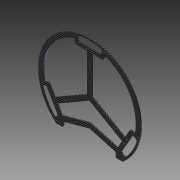
# Autodesk Inventor part: Middle Plate
Saved by Autodesk Inventor 2015 (Build 190159000, 159)
## iProperties
Created: 2016-08-09
Part Number: Middle Plate
Material: Polycarbonate, Clear
Document SubType Name: Modeling
Designer: James Yelland
Density: 1.2 g/cm^3
Appearance: Polycarbonate - Clear
Mass: 31.4673 g
Surface Area: 306.094 cm^2
Volume: 26.2228 cm^3
Author: James Yelland
Autodesk Inventor part; units mm, degrees
ref_plane "YZ Plane" through (0, 0, 0) normal (1, 0, 0) x (0, 1, 0)
ref_plane "XZ Plane" through (0, 0, 0) normal (0, 1, 0) x (-1, 0, 0)
ref_plane "XY Plane" through (0, 0, 0) normal (0, 0, 1) x (1, 0, 0)
sketch "Sketch1" plane through (0, 0, 0) normal (0, 1, 0) x (-1, 0, 0)
  circle A0 centre (-51.9527, -30.0153) radius 1.6
  circle A1 centre (0, 60) radius 1.6
  circle A2 centre (51.9527, -30.0153) radius 1.6
  line L0 (-76.2102, -44) -> (-65.7102, -62.1865)
  line L1 (-67.1743, -67.6506) -> (-69.6351, -69.0713)
  line L2 (-94.6351, -25.7701) -> (-92.1743, -24.3494)
  line L3 (-86.7102, -25.8135) -> (-76.2102, -44)
  arc A3 (-96.4496, -30.438) -> (-74.5849, -68.3088) centre (0, 0) ccw
  arc A4 (-94.6351, -25.7701) -> (-96.4496, -30.438) centre (-92.6351, -29.2342) ccw
  arc A5 (-86.7102, -25.8135) -> (-92.1743, -24.3494) centre (-90.1743, -27.8135) ccw
  arc A6 (-67.1743, -67.6506) -> (-65.7102, -62.1865) centre (-69.1743, -64.1865) ccw
  arc A7 (-74.5849, -68.3088) -> (-69.6351, -69.0713) centre (-71.6351, -65.6072) ccw
  line L4 (65.7102, -62.1865) -> (76.2102, -44)
  arc A8 (74.5849, -68.3088) -> (96.4496, -30.438) centre (0, 0) ccw
  arc A9 (65.7102, -62.1865) -> (67.1743, -67.6506) centre (69.1743, -64.1865) ccw
  line L5 (69.6351, -69.0713) -> (67.1743, -67.6506)
  arc A10 (69.6351, -69.0713) -> (74.5849, -68.3088) centre (71.6351, -65.6072) ccw
  arc A11 (92.1743, -24.3494) -> (86.7102, -25.8135) centre (90.1743, -27.8135) ccw
  line L6 (92.1743, -24.3494) -> (94.6351, -25.7701)
  arc A12 (96.4496, -30.438) -> (94.6351, -25.7701) centre (92.6351, -29.2342) ccw
  line L7 (76.2102, -44) -> (86.7102, -25.8135)
  line L8 (21, 88) -> (0, 88)
  arc A13 (21.8647, 98.7468) -> (-21.8647, 98.7468) centre (0, 0) ccw
  arc A14 (21, 88) -> (25, 92) centre (21, 92) ccw
  line L9 (25, 94.8414) -> (25, 92)
  arc A15 (25, 94.8414) -> (21.8647, 98.7468) centre (21, 94.8414) ccw
  arc A16 (-25, 92) -> (-21, 88) centre (-21, 92) ccw
  line L10 (-25, 92) -> (-25, 94.8414)
  arc A17 (-21.8647, 98.7468) -> (-25, 94.8414) centre (-21, 94.8414) ccw
  line L11 (0, 88) -> (-21, 88)
  line L12 (-75.1122, -39.9019) -> (-77.6122, -35.5718)
  line L13 (-77.6122, -35.5718) -> (-75.8801, -34.5718)
  line L14 (-75.8801, -34.5718) -> (-73.3801, -38.9019)
  line L15 (-73.3801, -38.9019) -> (-75.1122, -39.9019)
  line L16 (-70.3801, -44.0981) -> (-72.1122, -45.0981)
  line L17 (-67.8801, -48.4282) -> (-70.3801, -44.0981)
  line L18 (-69.6122, -49.4282) -> (-67.8801, -48.4282)
  line L19 (-72.1122, -45.0981) -> (-69.6122, -49.4282)
  line L20 (70.3801, -44.0981) -> (72.1122, -45.0981)
  line L21 (72.1122, -45.0981) -> (69.6122, -49.4282)
  line L22 (67.8801, -48.4282) -> (70.3801, -44.0981)
  line L23 (69.6122, -49.4282) -> (67.8801, -48.4282)
  line L24 (75.8801, -34.5718) -> (73.3801, -38.9019)
  line L25 (75.1122, -39.9019) -> (77.6122, -35.5718)
  line L26 (73.3801, -38.9019) -> (75.1122, -39.9019)
  line L27 (77.6122, -35.5718) -> (75.8801, -34.5718)
  line L28 (3, 83) -> (3, 85)
  line L29 (3, 85) -> (8, 85)
  line L30 (8, 83) -> (3, 83)
  line L31 (8, 85) -> (8, 83)
  line L32 (-8, 83) -> (-3, 83)
  line L33 (-3, 85) -> (-8, 85)
  line L34 (-3, 83) -> (-3, 85)
  line L35 (-8, 85) -> (-8, 83)
  line L36 (54.0074, -78) -> (54.0074, -71.5202)
  line L37 (52.5426, -69.5932) -> (0.5352, -55.1487)
  line L38 (-52.5426, -69.5932) -> (-0.5352, -55.1487)
  line L39 (-54.0074, -78) -> (-54.0074, -71.5202)
  arc A18 (68.5743, -79.5146) -> (-68.5743, -79.5146) centre (0, 0) ccw
  line L40 (67.2681, -80) -> (56.0074, -80)
  line L41 (-56.0074, -80) -> (-67.2681, -80)
  arc A19 (54.0074, -78) -> (56.0074, -80) centre (56.0074, -78) ccw
  arc A20 (67.2681, -80) -> (68.5743, -79.5146) centre (67.2681, -78) ccw
  arc A21 (54.0074, -71.5202) -> (52.5426, -69.5932) centre (52.0074, -71.5202) ccw
  arc A22 (0.5352, -55.1487) -> (-0.5352, -55.1487) centre (0, -57.0757) ccw
  arc A23 (-52.5426, -69.5932) -> (-54.0074, -71.5202) centre (-52.0074, -71.5202) ccw
  arc A24 (-56.0074, -80) -> (-54.0074, -78) centre (-56.0074, -78) ccw
  arc A25 (-68.5743, -79.5146) -> (-67.2681, -80) centre (-67.2681, -78) ccw
  line L42 (-30, 85) -> (-30, 87.3212)
  line L43 (30, 85) -> (30, 87.3212)
  arc A26 (-30, 85) -> (-25, 80) centre (-25, 85) ccw
  arc A27 (25, 80) -> (30, 85) centre (25, 85) ccw
  circle A28 centre (-30, 95.3939) radius 1.6
  circle A29 centre (30, 95.3939) radius 1.6
  arc A30 (-81.782, -18.3494) -> (-88.6122, -16.5192) centre (-86.1122, -20.8494) ccw
  line L44 (-88.6122, -16.5192) -> (-90.6224, -17.6799)
  circle A31 centre (-67.6136, -73.6777) radius 1.6
  circle A32 centre (-97.6136, -21.7162) radius 1.6
  arc A33 (88.6122, -16.5192) -> (81.782, -18.3494) centre (86.1122, -20.8494) ccw
  line L45 (88.6122, -16.5192) -> (90.6224, -17.6799)
  circle A34 centre (97.6136, -21.7162) radius 1.6
  circle A35 centre (67.6136, -73.6777) radius 1.6
  arc A36 (-32.6882, 89.1991) -> (-93.5928, -16.2908) centre (0, 0) ccw
  arc A37 (93.5928, -16.2908) -> (32.6882, 89.1991) centre (0, 0) ccw
  arc A38 (-30, 87.3212) -> (-32.6882, 89.1991) centre (-32, 87.3212) ccw
  arc A39 (32.6882, 89.1991) -> (30, 87.3212) centre (32, 87.3212) ccw
  arc A40 (90.6224, -17.6799) -> (93.5928, -16.2908) centre (91.6224, -15.9478) ccw
  arc A41 (-93.5928, -16.2908) -> (-90.6224, -17.6799) centre (-91.6224, -15.9478) ccw
  arc A42 (-57.9945, -59.5505) -> (-55.7273, -60.4776) centre (-56.2625, -58.5505) ccw
  arc A43 (55.7273, -60.4776) -> (57.9945, -59.5505) centre (56.2625, -58.5505) ccw
  arc A44 (-6, 2.3094) -> (-5, 4.0415) centre (-7, 4.0415) ccw
  arc A45 (5, 4.0415) -> (6, 2.3094) centre (7, 4.0415) ccw
  arc A46 (1, -6.3509) -> (-1, -6.3509) centre (0, -8.0829) ccw
  line L46 (-81.782, -18.3494) -> (-72.782, -33.9378)
  line L47 (-65.782, -46.0622) -> (-57.9945, -59.5505)
  line L48 (57.9945, -59.5505) -> (65.782, -46.0622)
  line L49 (72.782, -33.9378) -> (81.782, -18.3494)
  line L50 (-25, 80) -> (-7, 80)
  arc A47 (-65.05, -43.3301) -> (-65.782, -46.0622) centre (-64.05, -45.0622) ccw
  arc A48 (-72.782, -33.9378) -> (-70.05, -34.6699) centre (-71.05, -32.9378) ccw
  arc A49 (65.782, -46.0622) -> (65.05, -43.3301) centre (64.05, -45.0622) ccw
  arc A50 (70.05, -34.6699) -> (72.782, -33.9378) centre (71.05, -32.9378) ccw
  line L51 (7, 80) -> (25, 80)
  line L52 (5, 78) -> (5, 4.0415)
  line L53 (-5, 4.0415) -> (-5, 78)
  line L54 (-6, 2.3094) -> (-70.05, -34.6699)
  line L55 (-65.05, -43.3301) -> (-1, -6.3509)
  line L56 (65.05, -43.3301) -> (1, -6.3509)
  line L57 (70.05, -34.6699) -> (6, 2.3094)
  line L58 (0.5352, -45.1486) -> (55.7273, -60.4776)
  line L59 (-0.5352, -45.1486) -> (-55.7273, -60.4776)
  arc A51 (0.5352, -45.1486) -> (-0.5352, -45.1486) centre (0, -47.0757) ccw
  arc A52 (7, 80) -> (5, 78) centre (7, 78) ccw
  arc A53 (-5, 78) -> (-7, 80) centre (-7, 78) ccw
  point P0 (-63.7102, -65.6506)
  point P1 (-72.3705, -70.6506)
  point P2 (-97.3705, -27.3494)
  point P3 (88.7102, -22.3494)
  point P4 (97.3705, -27.3494)
  point P5 (-25, 88)
  point P6 (-25, 98)
  point P7 (68.0074, -80)
  point P8 (-68.0074, -80)
  point P9 (-30, 80)
  point P10 (-30, 90.1388)
  point P11 (30, 80)
  point P12 (30, 90.1388)
  point P13 (-84.282, -14.0192)
  point P14 (-93.0625, -19.0886)
  point P15 (84.282, -14.0192)
  point P16 (93.0625, -19.0886)
  point P17 (71.782, -35.6699)
  point P18 (66.782, -44.3301)
  point P19 (5, 80)
  point P20 (-5, 80)
  point P21 (-71.782, -35.6699)
  point P22 (-66.782, -44.3301)
  dimension "d45" = 360
  dimension "d46" = 360
  dimension "d126" = 360
  dimension "d121" = 2
  dimension "d122" = 2
  dimension "d123" = 2
  dimension "d124" = 2
  dimension "d128" = 2
  constraints: 120 end point, 100 point on circle, 54 centre point, 28 point on line, 18 tangent, 11 equal radius, 3 parallel, 2 coincident, 2 collinear, 2 horizontal, 1 vertical, 7 other
  measures "d121" radius of A38
  measures "d122" radius of A42
  measures "d123" radius of A44
  measures "d124" radius of A47
  measures "d128" radius of A51
extrude "Extrusion1" add sketch "Sketch1" along normal blind 2.5
body "Solid1"
